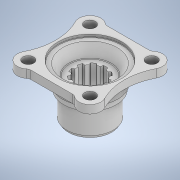
# Autodesk Inventor part: Деталь7
Saved by Autodesk Inventor 2021 (Build 250183000, 183)
## iProperties
Created: 2021-03-19
Part Number: Деталь7
Material: Типовые
Document SubType Name: Modeling
Designer: Данил
Density: 1 g/cm^3
Appearance: По умолчанию
Author: Данил
Autodesk Inventor part; units mm, degrees
ref_plane "YZ Plane" through (0, 0, 0) normal (1, 0, 0) x (0, 1, 0)
ref_plane "XZ Plane" through (0, 0, 0) normal (0, 1, 0) x (-1, 0, 0)
ref_plane "XY Plane" through (0, 0, 0) normal (0, 0, 1) x (1, 0, 0)
sketch "Эскиз1" plane through (0, 0, 0) normal (0, 0, 1) x (1, 0, 0)
  line L0 (0, 28.5) -> (0, -28.5)
  line L1 (17.5, -28.5) -> (23.7679, -28.5)
  line L2 (25.5, -25.5) -> (25.5, 0.5)
  line L3 (17.5, -28.5) -> (17.5, 13.5)
  line L4 (25.5, -25.5) -> (23.7679, -28.5)
  line L5 (25.5, 0.5) -> (29, 0.5)
  line L6 (29, 0.5) -> (29, 6.5)
  line L7 (29, 6.5) -> (30.5, 6.5)
  line L8 (17.5, 13.5) -> (22.4226, 13.5)
  line L9 (29.9282, 25.5) -> (34.5, 25.5)
  line L10 (35, 26) -> (35, 28.5)
  arc A0 (34.5, 25.5) -> (35, 26) centre (34.5, 26) ccw
  line L11 (23.2887, 14) -> (29.9282, 25.5)
  line L12 (35, 28.5) -> (60, 28.5)
  line L13 (60, 28.5) -> (60, 19.5)
  arc A1 (36, 18) -> (30.5, 6.5) centre (45.2727, 6.5) ccw
  line L14 (36, 18) -> (36, 18.5)
  line L15 (37, 19.5) -> (60, 19.5)
  arc A2 (22.4226, 13.5) -> (23.2887, 14) centre (22.4226, 14.5) ccw
  arc A3 (37, 19.5) -> (36, 18.5) centre (37, 18.5) ccw
  point P0 (0, 0)
  point P1 (0, 0)
  point P2 (25.5, -28.5)
  point P3 (23, 13.5)
  dimension "d0" = 57
  dimension "d1" = 35
  dimension "d2" = 51
  dimension "d3" = 3
  dimension "d4" = 30
  dimension "d5" = 58
  dimension "d6" = 61
  dimension "d7" = 35
  dimension "d8" = 6
  dimension "d12" = 3
  dimension "d13" = 0.5
  dimension "d14" = 30
  dimension "d15" = 46
  dimension "d16" = 15
  dimension "d17" = 70
  dimension "d18" = 1.5
  dimension "d19" = 9
  dimension "d20" = 72
  dimension "d21" = 120
  dimension "d22" = 1
  constraints: 32 end point, 8 point on circle, 6 tangent, 5 horizontal, 5 perpendicular, 4 centre point, 4 point on line, 4 vertical, 2 horizontal alignment, 1 coincident, 1 equal radius, 1 line through centre, 1 midpoint
  measures "d0" distance of L0.start L0.end
  measures "d1" diameter of L3 L0
  measures "d2" diameter of L2 L0
  measures "d3" distance of L2.start point (25.5, -28.5)
  measures "d4" angle of L2 L4
  measures "d5" diameter of L6 L0
  measures "d6" diameter of L7.end L0
  measures "d7" distance from line of L0.end L7
  measures "d8" distance between parallel lines of L5 L7
  measures "d12" distance from line of L9 L10.end
  measures "d13" radius of A0
  measures "d14" angle of L0 L11
  measures "d15" diameter of point (23, 13.5) L0
  measures "d16" distance from line of L8 L10.end
  measures "d17" diameter of L10.end L0
  measures "d18" distance from line of L14.start L15
  measures "d19" distance of L12.end L13.end
  measures "d20" diameter of L14 L0
  measures "d21" diameter of L13 L0
  measures "d22" radius of A2
revolve "Вращение1" add sketch "Эскиз1" angle 360 about axis through (0, 28.5, 0) along (0, -1, 0)
sketch "Эскиз2" plane through (0, 28.5, 0) normal (0, 1, 0) x (1, 0, 0)
  circle A0 centre (0, 0) radius 48 construction
  circle A1 centre (-33.9411, 33.9411) radius 6
  line L0 (0, 0) -> (0, 48) construction
  line L1 (0, 0) -> (-33.9411, 33.9411) construction
  circle A2 centre (33.9411, 33.9411) radius 6
  circle A3 centre (33.9411, -33.9411) radius 6
  circle A4 centre (-33.9411, -33.9411) radius 6
  dimension "d24" = 96
  dimension "d25" = 12
  dimension "d26" = 45
  constraints: 5 centre point, 5 point on circle, 4 end point, 3 equal radius, 2 horizontal alignment, 1 coincident, 1 vertical, 1 vertical alignment
  measures "d24" diameter of A0
  measures "d25" diameter of A1
  measures "d26" angle of L1 L0
extrude "Выдавливание1" cut sketch "Эскиз2" against normal through all
sketch "Эскиз3" plane through (0, 28.5, 0) normal (0, 1, 0) x (1, 0, 0)
  arc A0 (-37.7317, 0) -> (-44.6147, 28.457) centre (-100, 0) ccw
  circle A1 centre (-33.9411, 33.9411) radius 6 projected
  circle A2 centre (0, 0) radius 60 projected
  arc A3 (-25.0499, 42) -> (-44.6147, 28.457) centre (-33.9411, 33.9411) ccw
  line L0 (-25.0499, 42) -> (0, 42)
  line L1 (-37.7317, 0) -> (-60, 0)
  line L2 (0, 42) -> (0, 60)
  point P0 (0, 0)
  point P1 (-42.4264, 42.4264)
  dimension "d30" = 12
  dimension "d31" = 100
  dimension "d32" = 42
  constraints: 6 end point, 6 point on circle, 2 centre point, 2 horizontal, 2 horizontal alignment, 1 coincident, 1 perpendicular, 1 tangent, 1 vertical alignment
  measures "d30" radius of A3
  measures "d31" distance of A0.centre point (0, 0)
  measures "d32" distance from line of point (0, 0) L0
extrude "Выдавливание2" cut sketch "Эскиз3" against normal through all contours L1 A2 A3 A0 | A2 L2 L0 A3
mirror "Зеркальное отражение1" about plane through (0, 0, 0) normal (1, 0, 0) of "Выдавливание2"
mirror "Зеркальное отражение2" about plane through (0, 0, 0) normal (0, 0, 1) of "Выдавливание2", "Зеркальное отражение1"
fillet "Сопряжение1" radius 5 4 edges at (-25.0499, 24, -42) (25.0499, 24, -42) (-25.0499, 24, 42) (25.0499, 24, 42)
sketch "Эскиз4" plane through (0, 13.5, 0) normal (0, 1, 0) x (1, 0, 0)
  circle A0 centre (0, 0) radius 17.5 projected
  line L0 (-2.5, -17.3205) -> (2.5, -17.3205) construction
  circle A1 centre (0, 0) radius 15
  line L1 (-12.2033, -12.5431) -> (-8.1582, -15.482) construction
  line L2 (-17.2453, -2.9747) -> (-15.7002, -7.73) construction
  line L3 (-15.7002, 7.73) -> (-17.2453, 2.9747) construction
  line L4 (-8.1582, 15.482) -> (-12.2033, 12.5431) construction
  line L5 (2.5, 17.3205) -> (-2.5, 17.3205) construction
  line L6 (12.2033, 12.5431) -> (8.1582, 15.482) construction
  line L7 (17.2453, 2.9747) -> (15.7002, 7.73) construction
  line L8 (15.7002, -7.73) -> (17.2453, -2.9747) construction
  line L9 (8.1582, -15.482) -> (12.2033, -12.5431) construction
  line L10 (-8.1582, -15.482) -> (-6.2476, -13.637)
  line L11 (-2.5, -17.3205) -> (-2.9612, -14.7048)
  line L12 (-15.7002, -7.73) -> (-13.07, -7.3603)
  line L13 (-12.2033, -12.5431) -> (-11.0389, -10.1559)
  line L14 (-17.2453, 2.9747) -> (-14.9002, 1.7277)
  line L15 (-17.2453, -2.9747) -> (-14.9002, -1.7277)
  line L16 (-12.2033, 12.5431) -> (-11.0389, 10.1559)
  line L17 (-15.7002, 7.73) -> (-13.07, 7.3603)
  line L18 (-2.5, 17.3205) -> (-2.9612, 14.7048)
  line L19 (-8.1582, 15.482) -> (-6.2476, 13.637)
  line L20 (8.1582, 15.482) -> (6.2476, 13.637)
  line L21 (2.5, 17.3205) -> (2.9612, 14.7048)
  line L22 (15.7002, 7.73) -> (13.07, 7.3603)
  line L23 (12.2033, 12.5431) -> (11.0389, 10.1559)
  line L24 (17.2453, -2.9747) -> (14.9002, -1.7277)
  line L25 (17.2453, 2.9747) -> (14.9002, 1.7277)
  line L26 (12.2033, -12.5431) -> (11.0389, -10.1559)
  line L27 (15.7002, -7.73) -> (13.07, -7.3603)
  line L28 (2.5, -17.3205) -> (2.9612, -14.7048)
  line L29 (8.1582, -15.482) -> (6.2476, -13.637)
  point P0 (0, 0)
  point P1 (0, -17.3205)
  point P2 (-10.1807, -14.0126)
  point P3 (-16.4728, -5.3523)
  point P4 (-16.4728, 5.3523)
  point P5 (-10.1807, 14.0126)
  point P6 (0, 17.3205)
  point P7 (10.1807, 14.0126)
  point P8 (16.4728, 5.3523)
  point P9 (16.4728, -5.3523)
  point P10 (10.1807, -14.0126)
  point P11 (2.9612, 14.7048)
  dimension "d36" = 5
  dimension "d37" = 30
  dimension "d40" = 360
  dimension "d42" = 100
  dimension "d44" = 100
  dimension "d47" = 360
  constraints: 60 end point, 4 point on circle, 1 centre point, 1 coincident, 1 horizontal, 1 midpoint, 1 vertical alignment, 102 other
  measures "d36" distance of L0.start L0.end
  measures "d37" diameter of A1
  measures "d42" angle of L0 L11
  measures "d44" angle of L1 L10
extrude "Выдавливание3" add sketch "Эскиз4" against normal up to surface (42 mm away) contours A0 L24 A1 L25 | L22 A1 L23 A0 | A0 L26 A1 L27 | L20 A1 L21 A0 | A0 L28 A1 L29 | L18 A1 L19 A0 | A0 L10 A1 L11 | L16 A1 L17 A0 | A0 L12 A1 L13 | L14 A1 L15 A0
fillet "Сопряжение2" radius 0.3 20 edges at (15.7002, -7.5, 7.73) (8.1582, -7.5, 15.482) (2.5, -7.5, 17.3205) (12.2033, -7.5, 12.5431) (-2.5, -7.5, 17.3205) (-8.1582, -7.5, 15.482) (-12.2033, -7.5, 12.5431) (-15.7002, -7.5, 7.73) (-17.2453, -7.5, 2.9747) (-17.2453, -7.5, -2.9747) (-12.2033, -7.5, -12.5431) (-15.7002, -7.5, -7.73) (-2.5, -7.5, -17.3205) (-8.1582, -7.5, -15.482) (8.1582, -7.5, -15.482) (2.5, -7.5, -17.3205) (15.7002, -7.5, -7.73) (17.2453, -7.5, -2.9747) (12.2033, -7.5, -12.5431) (17.2453, -7.5, 2.9747)
sketch "Эскиз5" plane through (0, 0, 0) normal (0, 0, 1) x (1, 0, 0)
  line L0 (-23.7679, -28.5) -> (23.7679, -28.5) projected
  line L1 (15, -28.5) -> (15, 13.5) projected
  line L2 (17.5, -28.5) -> (15, -27.0566)
  line L3 (-35, 28.5) -> (35, 28.5) projected
  line L4 (23.0569, 28.5) -> (-23.0569, 28.5) projected
  line L5 (0, 28.5) -> (0, -28.5)
  point P0 (0, 0)
  dimension "d53" = 30
  dimension "d54" = 35
  constraints: 4 end point, 2 midpoint, 2 point on line
  measures "d53" angle of L0 L2
  measures "d54" diameter of L2.start L5
revolve "Вращение2" cut sketch "Эскиз5" angle 360 about axis through (0, 28.5, 0) along (0, -1, 0)
